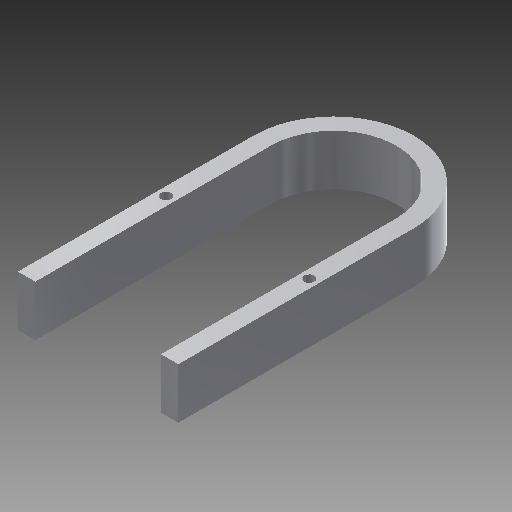
# Autodesk Inventor part: U
Saved by Autodesk Inventor 2018 (Build 220112000, 112)
## iProperties
Created: 2013-03-01
Part Number: U
Material: PVC-U
Document SubType Name: Modeling
Designer: Neef
Mass: 19.5415 g
Surface Area: 77.173 cm^2
Volume: 13.9582 cm^3
Density: 1.4 g/cm^3
Appearance: Smooth - White
Author: Neef
Autodesk Inventor part; units mm, degrees
ref_plane "YZ Plane" through (0, 0, 0) normal (1, 0, 0) x (0, 1, 0)
ref_plane "XZ Plane" through (0, 0, 0) normal (0, 1, 0) x (-1, 0, 0)
ref_plane "XY Plane" through (0, 0, 0) normal (0, 0, 1) x (1, 0, 0)
sketch "Skizze1" plane through (0, 0, 0) normal (0, 0, 1) x (1, 0, 0)
  line L0 (0, 46.8161) -> (0, -86.5527) projected
  line L1 (-33.3161, 0) -> (5.5527, 0) projected
  line L2 (-23, -67.5) -> (-23, 0)
  arc A0 (0, 23) -> (-23, 0) centre (0, 0) ccw
  line L3 (-23, -67.5) -> (-18, -67.5)
  line L4 (-18, -67.5) -> (-18, 0)
  arc A1 (0, 18) -> (-18, 0) centre (0, 0) ccw
  line L5 (0, 23) -> (0, 18)
  dimension "d0" = 67.5
  dimension "d1" = 5
  dimension "d2" = 23
  dimension "d3" = 23
  constraints: 8 end point, 4 point on circle, 4 point on line, 2 centre point, 2 perpendicular, 1 coincident, 1 collinear, 1 tangent, 1 vertical
  measures "d0" distance of L2.start L2.end
  measures "d1" distance between parallel lines of L2 L4
  measures "d2" distance between parallel lines of L0 L2
  measures "d3" radius of A0
extrude "Extrusion1" add sketch "Skizze1" along normal blind 14.5 contours L0 A1 L1 A0 | L1 L4 L3 L2
hole "Bohrung1" at (-20.5, -27.5, 14.5) direction (0, 0, -1) diameter 3 end through all
mirror "Spiegeln2" about plane through (0, 23, 0) normal (1, 0, 0)
